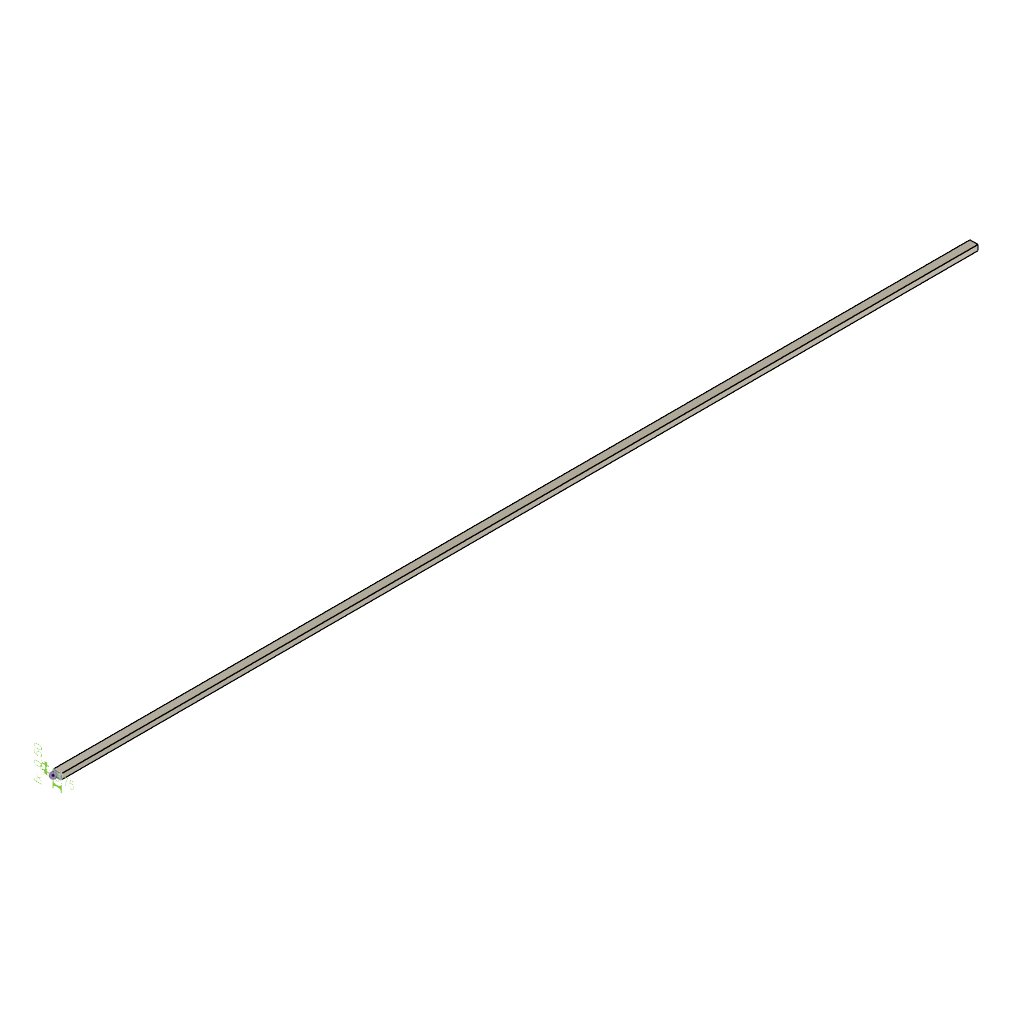
Tension_Study (Autodesk Fusion 360 design; units mm, degrees)
part number: 2026-09-09-17-24-20-586
Autodesk Fusion 360 part; units mm, degrees
sketch "Sketch1" plane through (0, 0, 0) normal (0, 1, 0) x (1, 0, 0)
  line L0 (0, 0) -> (19.05, 0)
  line L1 (19.05, 0) -> (19.05, -12.7)
  line L2 (19.05, -12.7) -> (0, -12.7)
  line L3 (0, -12.7) -> (0, 0)
  dimension "d8" = 19.05
  dimension "d9" = 12.7
  constraint horizontal L0
  constraint vertical L1
  constraint horizontal L2
  constraint vertical L3
  constraint coincident L0.start L3.end
  measures "d8" distance of L0.start L0.end
  measures "d9" distance of L0.start L2.end
extrude "Extrude1" add sketch "Sketch1" along normal blind 2143.125
equation "F_Load = 400 lbforce" comment "Load"
equation "E_Modulus = 10000000 psi" comment "Modulus"
equation "Delta = 0.009 in" comment "Max Deflection"
equation "Width = 0.75 in"
equation "Height = 0.5 in"
equation "Area = Width * Height"
equation "Length = Delta * Width * Height * E_Modulus / F_Load" comment "Area function wouldn't work"
equation "d8 = Width"
equation "d9 = Height"
equation "d10 = Length"
